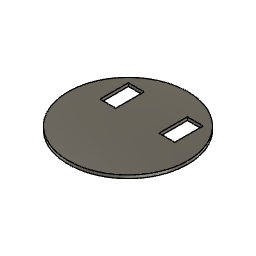
Robot assemblée v14 (Autodesk Fusion 360 archive; units mm, degrees)
design "Support robot"
Autodesk Fusion 360 part; units mm, degrees
sketch "Esquisse1" plane through (0, 0, 0) normal (0, 0, 1) x (1, 0, 0)
  circle A0 centre (0, 0) radius 95
  dimension "d1" = 190
  constraint coincident A0.centre origin
  measures "d1" diameter of A0
extrude "Extrusion1" add sketch "Esquisse1" along normal blind 5
sketch "Esquisse2" plane through (0, 0, 5) normal (0, 0, 1) x (-1, 0, 0)
  circle A0 centre (0, 0) radius 95
  line L0 (-34.3905, -60) -> (-59.3905, -60)
  line L1 (-59.3905, -60) -> (-59.3905, -15)
  line L2 (-59.3905, -15) -> (-34.3905, -15)
  line L3 (-34.3905, -15) -> (-34.3905, -60)
  line L4 (0, 95) -> (0, -95)
  line L5 (34.3905, -15) -> (34.3905, -60)
  line L6 (59.3905, -60) -> (59.3905, -15)
  line L7 (59.3905, -15) -> (34.3905, -15)
  line L8 (34.3905, -60) -> (59.3905, -60)
  dimension "d4" = 25
  dimension "d5" = 45
  constraint horizontal L0
  constraint vertical L1
  constraint horizontal L2
  constraint vertical L3
  constraint coincident A0 L4.start
  constraint coincident A0 L4.end
  constraint vertical L4
  constraint symmetric L0.start L4 L5.end
  constraint symmetric L0.end L4 L6.start
  constraint symmetric L1.end L4 L6.end
  constraint symmetric L2.end L4 L5.start
  measures "d4" distance of L0.start L0.end
  measures "d5" distance of L0.start L2.end
extrude "Extrusion2" cut sketch "Esquisse2" against normal blind 10 contours L0 L1 L2 L3 | L5 L6 L7 L8

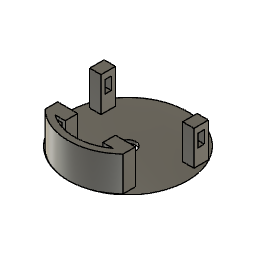
design "Socle dessus"
Autodesk Fusion 360 part; units mm, degrees
sketch "Esquisse1" plane through (0, 0, 0) normal (0, 0, 1) x (1, 0, 0)
  circle A0 centre (0, 0) radius 95
  circle A1 centre (0, 0) radius 12.5
  dimension "d1" = 190
  dimension "d2" = 25
  constraint coincident A0.centre A1.centre
  measures "d1" diameter of A0
  measures "d2" diameter of A1
extrude "Extrusion1" add sketch "Esquisse1" along normal blind 5
sketch "Esquisse2" plane through (0, 0, 5) normal (0, 0, 1) x (-1, 0, 0)
  circle A0 centre (0, 0) radius 12.5
  circle A1 centre (0, 0) radius 95
  line L0 (30, 50) -> (30, 70)
  line L1 (-65, -45) -> (-83, -45)
  line L2 (30, 70) -> (62, 70)
  line L3 (-30, 70) -> (-62, 70)
  line L4 (0, -1.75) -> (0, -22.5)
  line L5 (-65, -22) -> (-65, -45)
  arc A2 (62, 70) -> (-62, 70) centre (0, 5.62) ccw
  circle A3 centre (0, 0) radius 17.5
  arc A4 (46, 70) -> (-46, 70) centre (0, 6.9667) ccw
  line L6 (65, -22) -> (65, -45)
  line L7 (65, -45) -> (83, -45)
  line L8 (1.75, 0) -> (22.5, 0)
  line L9 (-30, 50) -> (-30, 70)
  line L10 (-62, 70) -> (-62, 50)
  line L11 (-83, -22) -> (-65, -22)
  line L12 (62, 70) -> (62, 50)
  circle A5 centre (0, 0) radius 95
  line L13 (-83, -45) -> (-83, -22)
  line L14 (83, -45) -> (83, -22)
  line L15 (62, 50) -> (30, 50)
  line L16 (-62, 50) -> (-30, 50)
  line L17 (83, -22) -> (65, -22)
  dimension "d125" = 65
  dimension "d126" = 22
  dimension "d127" = 23
  dimension "d128" = 18
  dimension "d129" = 20
  dimension "d130" = 32
  dimension "d131" = 50
  dimension "d132" = 30
  constraint horizontal L11
  constraint vertical L5
  constraint horizontal L1
  constraint vertical L13
  constraint symmetric L11.start L14.end L4
  constraint symmetric L6.start L5.start L4
  constraint symmetric L6.end L1.start L4
  constraint symmetric L1.end L7.end L4
  constraint horizontal L16
  constraint vertical L9
  constraint horizontal L3
  constraint vertical L10
  constraint symmetric L10.end L12.end L4
  constraint symmetric L9.start L0.start L4
  constraint symmetric L3.start L0.end L4
  constraint symmetric L2.end L3.end L4
  constraint tangent A2 A5
  constraint midpoint A4.start L2
  constraint midpoint A4.end L3
  measures "d125" distance of L4 L5
  measures "d126" distance of L8 L11
  measures "d127" distance of L1 L11
  measures "d128" distance of L5 L13
  measures "d129" distance of L3 L16
  measures "d130" distance of L9 L10
  measures "d131" distance of L8 L16
  measures "d132" distance of L4 L9
extrude "Extrusion2" add sketch "Esquisse2" along normal blind 55 contours L2 L3 A2 A4 | L0 L2 L12 L15 | L3 L9 L10 L16 | L1 L5 L11 L13 | L6 L7 L14 L17
fillet "Congé1" radius 95 1 edges at (-88.5711, -34.3535, 0)
sketch "Esquisse3" plane through (83, 0, 0) normal (1, 0, 0) x (0, 1, 0)
  line L0 (22, 5) -> (45, 5)
  line L1 (45, 5) -> (45, 60)
  line L2 (45, 60) -> (22, 60)
  line L3 (22, 60) -> (22, 5)
  line L4 (28.5, 50) -> (38.5, 50)
  line L5 (38.5, 50) -> (38.5, 30)
  line L6 (38.5, 30) -> (28.5, 30)
  line L7 (28.5, 30) -> (28.5, 50)
  dimension "d17" = 10
  dimension "d18" = 6.5
  dimension "d19" = 20
  constraint horizontal L4
  constraint vertical L5
  constraint horizontal L6
  constraint vertical L7
  measures "d17" distance of L5 L7
  measures "d18" distance of L3 L7
  measures "d19" distance of L4 L6
extrude "Extrusion3" cut sketch "Esquisse3" against normal blind 30 contours L4 L5 L6 L7
sketch "Esquisse4" plane through (-65, 0, 0) normal (1, 0, 0) x (0, 1, 0)
  line L0 (22, 5) -> (45, 5)
  line L1 (45, 5) -> (45, 60)
  line L2 (45, 60) -> (22, 60)
  line L3 (22, 60) -> (22, 5)
  line L4 (28.5, 50) -> (38.5, 50)
  line L5 (38.5, 50) -> (38.5, 30)
  line L6 (38.5, 30) -> (28.5, 30)
  line L7 (28.5, 30) -> (28.5, 50)
  dimension "d22" = 10
  dimension "d23" = 6.5
  dimension "d24" = 20
  dimension "d25" = 10
  constraint horizontal L4
  constraint vertical L5
  constraint horizontal L6
  constraint vertical L7
  measures "d22" distance of L5 L7
  measures "d23" distance of L3 L7
  measures "d24" distance of L4 L6
  measures "d25" distance of L2 L4
extrude "Extrusion4" cut sketch "Esquisse4" against normal blind 40 contours L4 L5 L6 L7
sketch "Esquisse5" plane through (0, -50, 0) normal (0, 1, 0) x (-1, 0, 0)
  line L0 (-62, 5) -> (-30, 5)
  line L1 (-30, 5) -> (-30, 60)
  line L2 (-30, 60) -> (-62, 60)
  line L3 (-62, 60) -> (-62, 5)
  line L4 (-50, 55) -> (-35, 55)
  line L5 (-35, 55) -> (-35, 35)
  line L6 (-35, 35) -> (-50, 35)
  line L7 (-50, 35) -> (-50, 55)
  arc A0 through (46, 60, -20) (0, 60, -35) (-46, 60, -20)
  line L8 (35, 55) -> (50, 55)
  line L9 (50, 55) -> (50, 35)
  line L10 (50, 35) -> (35, 35)
  line L11 (35, 35) -> (35, 55)
  line L12 (30, 5) -> (30, 60)
  line L13 (30, 60) -> (62, 60)
  point P0 (-30, 5)
  point P1 (30, 5)
  dimension "d29" = 5
  dimension "d30" = 15
  dimension "d31" = 20
  dimension "d32" = 5
  dimension "d33" = 15
  dimension "d34" = 5
  dimension "d35" = 20
  dimension "d37" = 5
  constraint horizontal L4
  constraint vertical L5
  constraint horizontal L6
  constraint vertical L7
  constraint horizontal L8
  constraint vertical L9
  constraint horizontal L10
  constraint vertical L11
  measures "d29" distance of L2 L4
  measures "d30" distance of L5.end L6.end
  measures "d31" distance of L4.start L6.end
  measures "d32" distance of L1 L5
  measures "d33" distance of L8.start L8.end
  measures "d34" distance of L11 L12
  measures "d35" distance of L8.end L9.end
  measures "d37" distance of L8 L13
extrude "Extrusion5" cut sketch "Esquisse5" against normal blind 20 contours L4 L5 L6 L7 | L8 L9 L10 L11

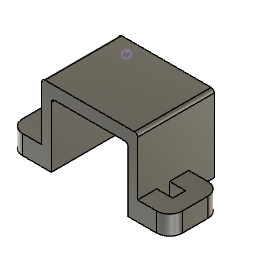
design "Support_Moteur"
Autodesk Fusion 360 part; units mm, degrees
sketch "Esquisse1" plane through (0, 0, 0) normal (0, 0, 1) x (1, 0, 0)
  line L0 (0, 0) -> (1.5, 0)
  line L1 (1.5, 0) -> (1.5, 1.2)
  line L2 (1.5, 1.2) -> (0, 1.2)
  line L3 (0, 1.2) -> (0, 0)
  dimension "d1" = 1.5
  dimension "d2" = 1.2
  constraint horizontal L0
  constraint vertical L1
  constraint horizontal L2
  constraint vertical L3
  constraint coincident L0.start L3.end
  measures "d1" distance of L0.start L0.end
  measures "d2" distance of L0.start L2.end
extrude "Extrusion1" add sketch "Esquisse1" along normal blind 1.2
sketch "Esquisse2" plane through (0, 0, 0) normal (0, 0, -1) x (1, 0, 0)
  line L0 (0, 0) -> (0, -1.2)
  line L1 (0, -1.2) -> (1.5, -1.2)
  line L2 (1.5, -1.2) -> (1.5, 0)
  line L3 (1.5, 0) -> (0, 0)
  line L4 (1.35, 0) -> (0.15, 0)
  line L5 (0.15, 0) -> (0.15, -1.2)
  line L6 (0.15, -1.2) -> (1.35, -1.2)
  line L7 (1.35, -1.2) -> (1.35, 0)
  line L8 (0.75, -1.2) -> (0.75, 0)
  dimension "d5" = 1.2
  dimension "d7" = 0.6
  constraint horizontal L4
  constraint vertical L5
  constraint horizontal L6
  constraint vertical L7
  constraint coincident L3 L4.start
  constraint midpoint L1 L8.start
  constraint midpoint L3 L8.end
  measures "d5" distance of L4.start L4.end
  measures "d7" distance of L7 L8
extrude "Extrusion2" cut sketch "Esquisse2" against normal blind 1 contours L1 L3 L4 L5 L6 L8 | L1 L3 L4 L6 L7 L8
sketch "Esquisse3" plane through (1.5, 0, 0) normal (1, 0, 0) x (0, 1, 0)
  line L0 (0, 0) -> (1.2, 0)
  line L1 (1.2, 0) -> (1.2, 1.2)
  line L2 (1.2, 1.2) -> (0, 1.2)
  line L3 (0, 1.2) -> (0, 0)
  line L4 (0, 0) -> (0.8, 0)
  line L5 (0.8, 0) -> (0.8, 0.3)
  line L6 (0.8, 0.3) -> (0, 0.3)
  line L7 (0, 0.3) -> (0, 0)
  dimension "d10" = 0.8
  dimension "d11" = 0.3
  constraint horizontal L4
  constraint vertical L5
  constraint horizontal L6
  constraint vertical L7
  constraint coincident L0.start L3.end
  measures "d10" distance of L0.start L4.end
  measures "d11" distance of L4 L6
extrude "Extrusion3" add sketch "Esquisse3" along normal blind 0.5 contours L0 L3 L4 L5 L6 L7
sketch "Esquisse4" plane through (0, 0, 0.3) normal (0, 0, 1) x (-1, 0, 0)
  line L0 (-1.5, -0.8) -> (-1.5, 0)
  line L1 (-1.5, 0) -> (-2, 0)
  line L2 (-2, 0) -> (-2, -0.8)
  line L3 (-2, -0.8) -> (-1.5, -0.8)
  line L4 (-1.5, -0.5) -> (-1.75, -0.5)
  line L5 (-1.75, -0.5) -> (-1.75, -0.3)
  line L6 (-1.75, -0.3) -> (-1.5, -0.3)
  line L7 (-1.5, -0.3) -> (-1.5, -0.5)
  line L8 (-1.5, -0.4) -> (-2, -0.4)
  dimension "d14" = 0.4
  dimension "d15" = 0.1
  dimension "d16" = 0.2
  dimension "d27" = 0.25
  constraint horizontal L4
  constraint vertical L5
  constraint horizontal L6
  constraint vertical L7
  constraint coincident L0 L4.start
  constraint coincident L0 L8.start
  constraint coincident L2 L8.end
  constraint perpendicular L2 L8
  measures "d14" distance of L3 L8
  measures "d15" distance of L6 L8
  measures "d16" distance of L4 L6
  measures "d27" distance of L5.end L6.end
extrude "Extrusion4" cut sketch "Esquisse4" against normal blind 0.5 contours L0 L4 L5 L7 L8 | L0 L5 L6 L7 L8
sketch "Esquisse5" plane through (0, 0, 0.3) normal (0, 0, 1) x (-1, 0, 0)
  line L0 (-1.75, -0.3) -> (-1.5, -0.3)
  line L1 (-1.5, -0.3) -> (-1.5, 0)
  line L2 (-1.5, 0) -> (-2, 0)
  line L3 (-2, 0) -> (-2, -0.8)
  line L4 (-2, -0.8) -> (-1.5, -0.8)
  line L5 (-1.5, -0.8) -> (-1.5, -0.5)
  line L6 (-1.5, -0.5) -> (-1.75, -0.5)
  line L7 (-1.75, -0.5) -> (-1.75, -0.3)
sketch "Esquisse6" plane through (0, 0, 0) normal (-1, 0, 0) x (0, -1, 0)
  line L0 (-1.2, 0) -> (0, 0)
  line L1 (0, 0) -> (0, 1.2)
  line L2 (0, 1.2) -> (-1.2, 1.2)
  line L3 (-1.2, 1.2) -> (-1.2, 0)
  line L4 (0, 0) -> (-0.8, 0)
  line L5 (-0.8, 0) -> (-0.8, 0.3)
  line L6 (-0.8, 0.3) -> (0, 0.3)
  line L7 (0, 0.3) -> (0, 0)
  dimension "d19" = 0.8
  dimension "d20" = 0.3
  constraint horizontal L4
  constraint vertical L5
  constraint horizontal L6
  constraint vertical L7
  constraint coincident L0.end L1.start
  measures "d19" distance of L0.end L4.end
  measures "d20" distance of L0.end L6.end
extrude "Extrusion5" add sketch "Esquisse6" along normal blind 0.5 contours L0 L1 L4 L5 L6 L7
sketch "Esquisse7" plane through (0, 0, 0.3) normal (0, 0, 1) x (-1, 0, 0)
  line L0 (0, 0) -> (0, -0.8)
  line L1 (0, -0.8) -> (0.5, -0.8)
  line L2 (0.5, -0.8) -> (0.5, 0)
  line L3 (0.5, 0) -> (0, 0)
  line L4 (0, -0.4) -> (0.5, -0.4)
  line L5 (0, -0.3) -> (0.25, -0.3)
  line L6 (0.25, -0.3) -> (0.25, -0.5)
  line L7 (0.25, -0.5) -> (0, -0.5)
  line L8 (0, -0.5) -> (0, -0.3)
  dimension "d23" = 0.25
  dimension "d24" = 0.2
  constraint midpoint L0 L4.start
  constraint midpoint L2 L4.end
  constraint horizontal L5
  constraint vertical L6
  constraint horizontal L7
  constraint vertical L8
  constraint coincident L0 L5.start
  measures "d23" distance of L5.start L5.end
  measures "d24" distance of L5.start L7.end
extrude "Extrusion6" cut sketch "Esquisse7" against normal blind 0.6 contours L0 L4 L5 L6 L8 | L0 L4 L6 L7 L8
fillet "Congé1" radius 0.2 4 edges at (2, 0, 0.15) (2, 0.8, 0.15) (-0.5, 0, 0.15) (-0.5, 0.8, 0.15)
fillet "Congé2" radius 0.05 2 edges at (1.5, 0.6, 1.2) (0, 0.6, 1.2)
fillet "Congé3" radius 0.05 2 edges at (1.35, 0.6, 1) (0.15, 0.6, 1)
scale "Echelle1" factor 10 about (0.05, 1.2, 1.2) bodies 1

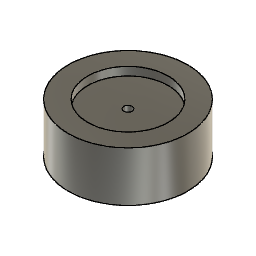
design "Roue"
Autodesk Fusion 360 part; units mm, degrees
sketch "Esquisse1" plane through (0, 0, 0) normal (0, 0, 1) x (1, 0, 0)
  circle A0 centre (0, 0) radius 2.15
  dimension "d1" = 4.3
  constraint coincident A0.centre origin
  measures "d1" diameter of A0
extrude "Extrusion1" add sketch "Esquisse1" along normal blind 1.8
sketch "Esquisse2" plane through (0, 0, 1.8) normal (0, 0, 1) x (-1, 0, 0)
  circle A0 centre (0, 0) radius 2.15
  circle A1 centre (0, 0) radius 1.45
  dimension "d4" = 2.9
  constraint concentric A0 A1
  measures "d4" diameter of A1
extrude "Extrusion2" cut sketch "Esquisse2" against normal blind 0.3 contours A1
sketch "Esquisse3" plane through (0, 0, 0) normal (0, 0, -1) x (1, 0, 0)
  circle A0 centre (0, 0) radius 2.15
  circle A1 centre (0, 0) radius 1.1
  dimension "d7" = 2.2
  constraint concentric A0 A1
  measures "d7" diameter of A1
extrude "Extrusion3" cut sketch "Esquisse3" against normal blind 0.5 contours A1
sketch "Esquisse4" plane through (0, 0, 1.5) normal (0, 0, 1) x (-1, 0, 0)
  circle A0 centre (0, 0) radius 1.45
  circle A1 centre (0, 0) radius 0.15
  dimension "d10" = 0.3
  constraint concentric A0 A1
  measures "d10" diameter of A1
extrude "Extrusion4" cut sketch "Esquisse4" against normal blind 3.8 contours A1
scale "Echelle1" factor 10 about (1.45, 0, 1.8) bodies 1

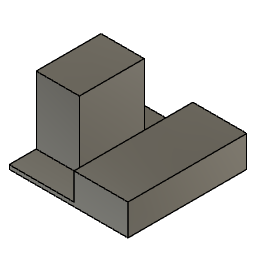
design "MotorDriver"
Autodesk Fusion 360 part; units mm, degrees
sketch "Esquisse1" plane through (0, 0, 0) normal (0, 0, 1) x (1, 0, 0)
  line L0 (0, 0) -> (4.4, 0)
  line L1 (4.4, 0) -> (4.4, 4.4)
  line L2 (4.4, 4.4) -> (0, 4.4)
  line L3 (0, 4.4) -> (0, 0)
  dimension "d1" = 4.4
  dimension "d2" = 4.4
  constraint horizontal L0
  constraint vertical L1
  constraint horizontal L2
  constraint vertical L3
  constraint coincident L0.start L3.end
  measures "d1" distance of L0.start L0.end
  measures "d2" distance of L0.start L2.end
extrude "Extrusion1" add sketch "Esquisse1" along normal blind 0.15
sketch "Esquisse2" plane through (0, 0, 0.15) normal (0, 0, 1) x (-1, 0, 0)
  line L0 (0, -4.4) -> (0, 0)
  line L1 (0, 0) -> (-4.4, 0)
  line L2 (-4.4, 0) -> (-4.4, -4.4)
  line L3 (-4.4, -4.4) -> (0, -4.4)
  line L4 (-4.4, 0) -> (-2.4, 0)
  line L5 (-2.4, 0) -> (-2.4, -4.4)
  line L6 (-2.4, -4.4) -> (-4.4, -4.4)
  line L7 (-4.4, -4.4) -> (-4.4, 0)
  dimension "d5" = 2
  constraint horizontal L4
  constraint vertical L5
  constraint horizontal L6
  constraint vertical L7
  constraint coincident L3 L5.end
  constraint coincident L1.end L2.start
  measures "d5" distance of L1.end L4.end
extrude "Extrusion2" add sketch "Esquisse2" along normal blind 1 contours L1 L2 L3 L4 L5 L6 L7
sketch "Esquisse3" plane through (0, 0, 0.15) normal (0, 0, 1) x (-1, 0, 0)
  line L0 (-2.4, 0) -> (-2.4, -4.4)
  line L1 (-2.4, -4.4) -> (0, -4.4)
  line L2 (0, -4.4) -> (0, 0)
  line L3 (0, 0) -> (-2.4, 0)
  line L4 (0, -3.4) -> (-1.6, -3.4)
  line L5 (-1.6, -3.4) -> (-1.6, -1)
  line L6 (-1.6, -1) -> (0, -1)
  line L7 (0, -1) -> (0, -3.4)
  dimension "d8" = 1.6
  dimension "d9" = 2.4
  dimension "d11" = 1
  constraint horizontal L4
  constraint vertical L5
  constraint horizontal L6
  constraint vertical L7
  constraint coincident L2 L4.start
  measures "d8" distance of L4.start L4.end
  measures "d9" distance of L4.start L6.end
  measures "d11" distance of L3 L6
extrude "Extrusion3" add sketch "Esquisse3" along normal blind 2.5 contours L2 L4 L5 L6 L7
scale "Echelle1" factor 10 about (0, 3.4, 2.65) bodies 1

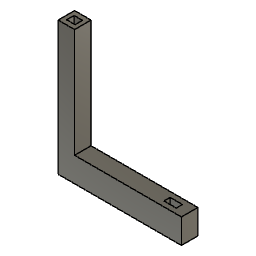
design "Bras moteur boule"
Autodesk Fusion 360 part; units mm, degrees
sketch "Esquisse1" plane through (0, 0, 0) normal (0, 0, 1) x (1, 0, 0)
  line L0 (0, 0) -> (8, 0)
  line L1 (8, 0) -> (8, 8)
  line L2 (8, 8) -> (0, 8)
  line L3 (0, 8) -> (0, 0)
  dimension "d1" = 8
  dimension "d2" = 8
  constraint horizontal L0
  constraint vertical L1
  constraint horizontal L2
  constraint vertical L3
  constraint coincident L0.start L3.end
  measures "d1" distance of L1.end L2.end
  measures "d2" distance of L0.start L2.end
extrude "Extrusion1" add sketch "Esquisse1" along normal blind 65
sketch "Esquisse8" plane through (0, 0, 65) normal (0, 0, 1) x (-1, 0, 0)
  line L0 (0, -8) -> (0, 0)
  line L1 (0, 0) -> (-8, 0)
  line L2 (-8, 0) -> (-8, -8)
  line L3 (-8, -8) -> (0, -8)
  line L4 (0, -4) -> (-8, -4)
  line L5 (-1.95, -4) -> (-6.05, -4)
  line L6 (-6.05, -4) -> (-6.05, -5.8)
  line L7 (-6.05, -5.8) -> (-1.95, -5.8)
  line L8 (-1.95, -5.8) -> (-1.95, -4)
  line L9 (-4, -8) -> (-4, 0)
  line L10 (-1.95, -2.2) -> (-1.95, -4)
  line L11 (-6.05, -2.2) -> (-1.95, -2.2)
  line L12 (-6.05, -4) -> (-6.05, -2.2)
  dimension "d41" = 4.1
  dimension "d42" = 2.05
  dimension "d43" = 1.8
  constraint midpoint L0 L4.start
  constraint midpoint L2 L4.end
  constraint horizontal L5
  constraint vertical L6
  constraint horizontal L7
  constraint vertical L8
  constraint coincident L4 L5.start
  constraint midpoint L3 L9.start
  constraint midpoint L1 L9.end
  constraint symmetric L8.end L5 L10.end
  constraint symmetric L6.start L5 L12.start
  constraint symmetric L6.end L5 L11.start
  constraint symmetric L7.end L5 L10.start
  measures "d41" distance of L6 L8
  measures "d42" distance of L8 L9
  measures "d43" distance of L5.start L7.end
extrude "Extrusion8" cut sketch "Esquisse8" against normal blind 6 contours L4 L5 L7 L8 L9 | L4 L5 L9 L10 L11 | L4 L5 L6 L7 L9 | L4 L5 L9 L11 L12
sketch "Esquisse9" plane through (8, 0, 0) normal (1, 0, 0) x (0, 1, 0)
  line L0 (0, 0) -> (8, 0)
  line L1 (8, 0) -> (8, 65)
  line L2 (8, 65) -> (0, 65)
  line L3 (0, 65) -> (0, 0)
  line L4 (0, 0) -> (8, 0)
  line L5 (8, 0) -> (8, 12)
  line L6 (8, 12) -> (0, 12)
  line L7 (0, 12) -> (0, 0)
  dimension "d46" = 12
  constraint horizontal L4
  constraint vertical L5
  constraint horizontal L6
  constraint vertical L7
  constraint coincident L1 L5.end
  constraint coincident L0.start L3.end
  measures "d46" distance of L4 L6
extrude "Extrusion9" add sketch "Esquisse9" along normal blind 52 contours L0 L1 L3 L4 L5 L6 L7
sketch "Esquisse10" plane through (0, 0, 12) normal (0, 0, 1) x (-1, 0, 0)
  line L0 (-8, -8) -> (-8, 0)
  line L1 (-8, 0) -> (-60, 0)
  line L2 (-60, 0) -> (-60, -8)
  line L3 (-60, -8) -> (-8, -8)
  line L4 (-55, -5.5) -> (-49, -5.5)
  line L5 (-49, -5.5) -> (-49, -2.5)
  line L6 (-49, -2.5) -> (-55, -2.5)
  line L7 (-55, -2.5) -> (-55, -5.5)
  dimension "d49" = 2.5
  dimension "d50" = 2.5
  dimension "d51" = 5
  dimension "d52" = 6
  constraint horizontal L4
  constraint vertical L5
  constraint horizontal L6
  constraint vertical L7
  measures "d49" distance of L3 L4
  measures "d50" distance of L1 L6
  measures "d51" distance of L2 L7
  measures "d52" distance of L5 L7
extrude "Extrusion10" cut sketch "Esquisse10" against normal blind 23 contours L4 L5 L6 L7

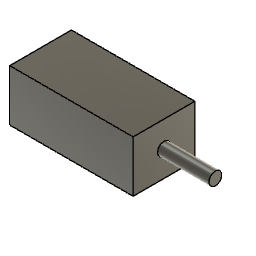
design "Moteur"
Autodesk Fusion 360 part; units mm, degrees
sketch "Esquisse1" plane through (0, 0, 0) normal (0, 0, 1) x (1, 0, 0)
  line L0 (0, 0) -> (2.4, 0)
  line L1 (2.4, 0) -> (2.4, 1.2)
  line L2 (2.4, 1.2) -> (0, 1.2)
  line L3 (0, 1.2) -> (0, 0)
  dimension "d1" = 2.4
  dimension "d2" = 1.2
  constraint horizontal L0
  constraint vertical L1
  constraint horizontal L2
  constraint vertical L3
  constraint coincident L0.start L3.end
  measures "d1" distance of L0.start L0.end
  measures "d2" distance of L0.end L2
extrude "Extrusion1" add sketch "Esquisse1" along normal blind 1
sketch "Esquisse2" plane through (2.4, 0, 0) normal (1, 0, 0) x (0, 1, 0)
  line L0 (0, 0) -> (1.2, 0)
  line L1 (1.2, 0) -> (1.2, 1)
  line L2 (1.2, 1) -> (0, 1)
  line L3 (0, 1) -> (0, 0)
  circle A0 centre (0.6, 0.5) radius 0.125
  dimension "d5" = 0.25
  measures "d5" diameter of A0
extrude "Extrusion2" add sketch "Esquisse2" along normal blind 1 contours A0
scale "Echelle1" factor 10 about (0, 1.2, 1) bodies 1

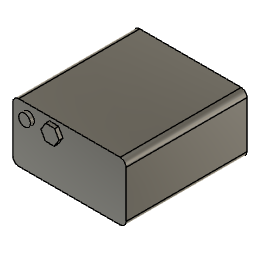
design "Bloc pile 12V"
Autodesk Fusion 360 part; units mm, degrees
sketch "Esquisse1" plane through (0, 0, 0) normal (0, 0, 1) x (1, 0, 0)
  line L0 (0, 0) -> (58, 0)
  line L1 (58, 0) -> (58, 62)
  line L2 (58, 62) -> (0, 62)
  line L3 (0, 62) -> (0, 0)
  dimension "d1" = 58
  dimension "d2" = 62
  constraint horizontal L0
  constraint vertical L1
  constraint horizontal L2
  constraint vertical L3
  constraint coincident L0.start L3.end
  measures "d1" distance of L0.start L0.end
  measures "d2" distance of L0.start L2.end
extrude "Extrusion1" add sketch "Esquisse1" along normal blind 30
fillet "Congé1" radius 3 4 edges at (58, 31, 30) (58, 31, 0) (0, 31, 30) (0, 31, 0)
sketch "Esquisse2" plane through (0, 0, 0) normal (0, -1, 0) x (1, 0, 0)
  arc A0 (0, 3) -> (3, 0) centre (3, 3) ccw
  line L0 (3, 0) -> (55, 0)
  arc A1 (55, 0) -> (58, 3) centre (55, 3) ccw
  line L1 (58, 3) -> (58, 27)
  arc A2 (58, 27) -> (55, 30) centre (55, 27) ccw
  line L2 (55, 30) -> (3, 30)
  arc A3 (3, 30) -> (0, 27) centre (3, 27) ccw
  line L3 (0, 27) -> (0, 3)
  circle A4 centre (8, 24) radius 3
  dimension "d7" = 6
  dimension "d8" = 6
  dimension "d9" = 8
  measures "d7" diameter of A4
  measures "d8" distance of L2 A4.centre
  measures "d9" distance of L3 A4.centre
sketch "Esquisse3" plane through (0, 0, 0) normal (0, -1, 0) x (1, 0, 0)
  line L0 (18.832, 28.0784) -> (16.384, 24.1616)
  line L1 (16.384, 24.1616) -> (18.552, 20.0833)
  line L2 (18.552, 20.0833) -> (23.168, 19.9216)
  line L3 (23.168, 19.9216) -> (25.616, 23.8384)
  line L4 (25.616, 23.8384) -> (23.448, 27.9167)
  line L5 (23.448, 27.9167) -> (18.832, 28.0784)
  line L6 (55, 30) -> (3, 30)
  line L7 (0, 27) -> (0, 3)
  point P0 (21, 24)
  dimension "d10" = 8
  dimension "d11" = 6
  dimension "d12" = 21
  measures "d10" distance of L2 L5
  measures "d11" distance of P0 L6
  measures "d12" distance of P0 L7
extrude "Extrusion2" add sketch "Esquisse2" sketch "Esquisse3" along normal blind 2 contours A4 of sketch 2

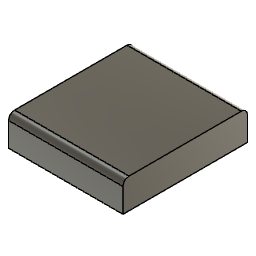
design "Bloc Pile 6v"
Autodesk Fusion 360 part; units mm, degrees
sketch "Esquisse1" plane through (0, 0, 0) normal (0, 0, 1) x (1, 0, 0)
  line L0 (0, 0) -> (57, 0)
  line L1 (57, 0) -> (57, 62)
  line L2 (57, 62) -> (0, 62)
  line L3 (0, 62) -> (0, 0)
  dimension "d1" = 57
  dimension "d2" = 62
  constraint horizontal L0
  constraint vertical L1
  constraint horizontal L2
  constraint vertical L3
  constraint coincident L0.start L3.end
  measures "d1" distance of L0.start L0.end
  measures "d2" distance of L0.start L2.end
extrude "Extrusion1" add sketch "Esquisse1" along normal blind 15
fillet "Congé1" radius 3 2 edges at (28.5, 62, 15) (28.5, 0, 15)

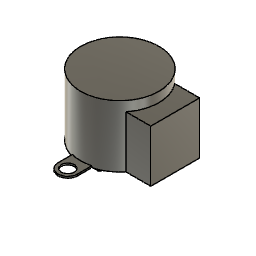
design "Moteur_Boule"
Autodesk Fusion 360 part; units mm, degrees
sketch "Esquisse1" plane through (0, 0, 0) normal (0, 0, 1) x (1, 0, 0)
  circle A0 centre (0, 0) radius 12
  line L0 (9, 0) -> (17, 0)
  line L1 (17, -7.5) -> (9, -7.5)
  line L2 (9, -7.5) -> (9, 7.5)
  line L3 (9, 7.5) -> (17, 7.5)
  line L4 (17, 7.5) -> (17, -7.5)
  dimension "d1" = 24
  dimension "d3" = 8
  dimension "d4" = 17
  dimension "d5" = 15
  dimension "d8" = 7.5
  dimension "d9" = 8
  constraint coincident A0.centre origin
  constraint horizontal L0
  constraint horizontal L1
  constraint vertical L2
  constraint horizontal L3
  constraint vertical L4
  constraint collinear A0.centre L0.start L0.end
  constraint collinear L0.end L1.start L3.end
  measures "d1" diameter of A0
  measures "d3" distance of L0.start L0.end
  measures "d4" distance of A0.centre L0.end
  measures "d5" distance of L1 L3
  measures "d8" distance of L0 L1
  measures "d9" distance of L2.end L3.end
extrude "Extrusion1" add sketch "Esquisse1" along normal blind 16
sketch "Esquisse2" plane through (0, 0, 16) normal (0, 0, 1) x (-1, 0, 0)
  arc A0 (-9.3675, -7.5) -> (-9.3675, 7.5) centre (0, 0) ccw
  line L0 (-9.3675, 7.5) -> (-17, 7.5)
  line L1 (-17, 7.5) -> (-17, -7.5)
  line L2 (-17, -7.5) -> (-9.3675, -7.5)
  circle A1 centre (0, 0) radius 12
  constraint concentric A0 A1
extrude "Extrusion2" add sketch "Esquisse2" along normal blind 3 contours A0 A1
sketch "Esquisse5" plane through (0, 0, 0) normal (0, 0, -1) x (1, 0, 0)
  arc A0 (9.3675, 7.5) -> (9.3675, -7.5) centre (0, 0) ccw
  line L0 (9.3675, -7.5) -> (17, -7.5)
  line L1 (17, -7.5) -> (17, 7.5)
  line L2 (17, 7.5) -> (9.3675, 7.5)
  circle A1 centre (0, 16) radius 2
  line L3 (0, 0) -> (12, 0)
  circle A2 centre (0, 0) radius 12
  line L4 (3, 16) -> (3, 11.619)
  line L5 (0, 0) -> (0, 19)
  arc A3 (-3, -16) -> (0, -19) centre (0, -16) ccw
  line L6 (3, -16) -> (3, -11.619)
  circle A4 centre (0, -16) radius 2
  line L7 (-3, 16) -> (-3, 11.619)
  arc A5 (0, -19) -> (3, -16) centre (0, -16) ccw
  arc A6 (0, 19) -> (-3, 16) centre (0, 16) ccw
  line L8 (-3, 16) -> (3, 16)
  arc A7 (3, 16) -> (0, 19) centre (0, 16) ccw
  line L9 (-3, -16) -> (-3, -11.619)
  point P0 (0, 12)
  dimension "d27" = 19
  dimension "d28" = 4
  dimension "d29" = 24
  dimension "d30" = 3
  constraint coincident A0.centre L3.start
  constraint vertical L5
  constraint coincident A1.centre L5
  constraint coincident P0 L5
  constraint perpendicular L3 L5
  constraint coincident A1.centre A6.centre
  constraint perpendicular L5 L8
  constraint coincident L4.end A2
  constraint tangent L4 A7
  constraint coincident L7.end A2
  constraint tangent L7 A6
  constraint perpendicular L7 L8
  constraint symmetric A3.end L5.end L3
  constraint symmetric A1 L3 A4
  constraint symmetric L6.start L4.start L3
  constraint symmetric L3 A5 A7
  constraint symmetric A3.start L7.start L3
  constraint symmetric L3 A3 A6
  constraint symmetric L4.end L6.end L3
  constraint symmetric L7.end L9.end L3
  measures "d27" distance of A0.centre L5.end
  measures "d28" diameter of A1
  measures "d29" diameter of A2
  measures "d30" distance of L8 A7
extrude "Extrusion4" add sketch "Esquisse5" against normal blind 0.5 contours A0 A1 A2 L4 L5 L8 | A0 A1 A2 L5 L7 L8 | A1 L5 L8 A7 | A1 L5 A6 L8 | A0 A2 A3 L6 A5 L9
sketch "Esquisse6" plane through (0, 0, 0) normal (0, 0, -1) x (1, 0, 0)
  circle A0 centre (0, -16) radius 2
  circle A1 centre (0, 16) radius 2
  arc A2 (3, -11.619) -> (9.3675, -7.5) centre (0, 0) ccw
  line L0 (9.3675, -7.5) -> (17, -7.5)
  line L1 (17, -7.5) -> (17, 7.5)
  line L2 (17, 7.5) -> (9.3675, 7.5)
  arc A3 (9.3675, 7.5) -> (3, 11.619) centre (0, 0) ccw
  line L3 (3, 11.619) -> (3, 16)
  arc A4 (3, 16) -> (-3, 16) centre (0, 16) ccw
  line L4 (-3, 16) -> (-3, 11.619)
  arc A5 (-3, 11.619) -> (-3, -11.619) centre (0, 0) ccw
  line L5 (-3, -11.619) -> (-3, -16)
  arc A6 (-3, -16) -> (3, -16) centre (0, -16) ccw
  line L6 (3, -16) -> (3, -11.619)
  circle A7 centre (-7, 0) radius 4
  line L7 (-7, 0) -> (-12, 0)
  dimension "d33" = 8
  dimension "d34" = 5
  constraint coincident A7.centre L7.start
  constraint midpoint A5 L7.end
  constraint horizontal L7
  measures "d33" diameter of A7
  measures "d34" distance of A7.centre L7.end
extrude "Extrusion5" add sketch "Esquisse6" along normal blind 1 contours A7
sketch "Esquisse7" plane through (0, 0, -1) normal (0, 0, -1) x (1, 0, 0)
  circle A0 centre (-7, 0) radius 4
  circle A1 centre (-7, 0) radius 2.5
  dimension "d37" = 5
  constraint concentric A0 A1
  measures "d37" diameter of A1
extrude "Extrusion6" add sketch "Esquisse7" along normal blind 9 contours A1
sketch "Esquisse8" plane through (0, 0, -10) normal (0, 0, -1) x (1, 0, 0)
  circle A0 centre (-7, 0) radius 2.5
  line L0 (-7, 0) -> (-9.5, 0)
  line L1 (-7, 0) -> (-4.5, 0)
  line L2 (-9, 0) -> (-5, 0)
  line L3 (-5, 0) -> (-5, 1.5)
  line L4 (-5, 1.5) -> (-9, 1.5)
  line L5 (-9, 1.5) -> (-9, 0)
  line L6 (-5, -1.5) -> (-9, -1.5)
  line L7 (-9, -1.5) -> (-9, 0)
  line L8 (-5, 0) -> (-5, -1.5)
  dimension "d43" = 4
  dimension "d44" = 1.5
  dimension "d45" = 2
  constraint coincident A0.centre L0.start
  constraint coincident A0 L0.end
  constraint horizontal L0
  constraint coincident A0 L1.end
  constraint parallel L0 L1
  constraint horizontal L2
  constraint vertical L3
  constraint horizontal L4
  constraint vertical L5
  constraint coincident L0 L2.start
  constraint symmetric L5.end L2 L7.end
  constraint symmetric L3.start L2 L8.start
  constraint symmetric L3.end L2 L6.start
  constraint symmetric L4.end L2 L6.end
  measures "d43" distance of L3.end L4.end
  measures "d44" distance of L1 L4
  measures "d45" distance of A0.centre L5
extrude "Extrusion7" cut sketch "Esquisse8" against normal blind 6 contours A0 L4 | A0 L6

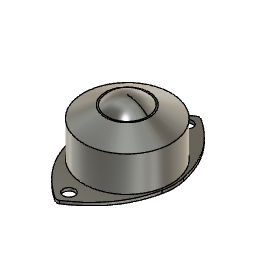
design "Roue Pivot"
Autodesk Fusion 360 part; units mm, degrees
sketch "Esquisse1" plane through (0, 0, 0) normal (0, 0, 1) x (1, 0, 0)
  circle A0 centre (0, 0) radius 16
  line L0 (0, 25) -> (0, -25)
  line L1 (0, 16) -> (0, 25)
  circle A1 centre (0, 20.5) radius 2
  spline S0 degree 5 poles (-15.998, 0.25) (-15.7389, 1.9932) (-15.1133, 5.2622) (-13.8531, 9.5141) (-11.6152, 14.0579) (-8.1767, 18.4749) (-5.0788, 21.3679) (-2.5998, 23.2801) (-0.8781, 24.445) (0, 25) knots 0 0 0 0 0 0 0.2 0.4 0.6 0.8 1 1 1 1 1 1
  line L2 (-16.6171, -3.9145) -> (-15.379, 4.4145)
  spline S1 degree 5 poles (15.998, 0.25) (15.7389, 1.9932) (15.1133, 5.2622) (13.8531, 9.5141) (11.6152, 14.0579) (8.1767, 18.4749) (5.0788, 21.3679) (2.5998, 23.2801) (0.8781, 24.445) (0, 25) knots 0 0 0 0 0 0 0.2 0.4 0.6 0.8 1 1 1 1 1 1
  line L3 (-2.0948, 23.676) -> (2.0948, 26.324)
  line L4 (16.6171, -3.9145) -> (15.379, 4.4145)
  line L5 (2.0948, 23.676) -> (-2.0948, 26.324)
  line L6 (-15.998, 0.25) -> (15.998, 0.25)
  spline S2 degree 5 poles (-15.998, 0.25) (-15.7389, -1.4932) (-15.1133, -4.7622) (-13.8531, -9.0141) (-11.6152, -13.5579) (-8.1767, -17.9749) (-5.0788, -20.8679) (-2.5998, -22.7801) (-0.8781, -23.945) (0, -24.5) knots 0 0 0 0 0 0 0.2 0.4 0.6 0.8 1 1 1 1 1 1
  line L7 (-16.6171, 4.4145) -> (-15.379, -3.9145)
  line L8 (-2.0948, -23.176) -> (2.0948, -25.824)
  spline S3 degree 5 poles (15.998, 0.25) (15.7389, -1.4932) (15.1133, -4.7622) (13.8531, -9.0141) (11.6152, -13.5579) (8.1767, -17.9749) (5.0788, -20.8679) (2.5998, -22.7801) (0.8781, -23.945) (0, -24.5) knots 0 0 0 0 0 0 0.2 0.4 0.6 0.8 1 1 1 1 1 1
  line L9 (16.6171, 4.4145) -> (15.379, -3.9145)
  line L10 (2.0948, -23.176) -> (-2.0948, -25.824)
  circle A2 centre (0, -20) radius 2
  point P0 (0, 16)
  dimension "d1" = 32
  dimension "d2" = 50
  dimension "d3" = 25
  dimension "d4" = 4
  constraint coincident A0.centre origin
  constraint vertical L0
  constraint coincident A0 P0
  constraint coincident L0 P0
  constraint midpoint L1 A1.centre
  constraint coincident A0 S0.start
  constraint midpoint S0.start L2
  constraint coincident A0 L2.end
  constraint midpoint L0.start L3
  constraint symmetric L1.end L0 S0.end
  constraint symmetric L0 P0 L1.start
  constraint symmetric L0 S0.start S1.start
  constraint symmetric L0 L2.start L4.start
  constraint symmetric L0 L2.end L4.end
  constraint symmetric L0 L3.start L5.start
  constraint symmetric L0 L3.end L5.end
  constraint symmetric L0.start L6 S2.end
  constraint symmetric A1 L6 A2
  constraint symmetric S0.start L6 S2.start
  constraint symmetric L2.start L6 L7.start
  constraint symmetric L2.end L6 L7.end
  constraint symmetric S1.start L6 S3.start
  constraint symmetric L3.start L6 L8.start
  constraint symmetric L3.end L6 L8.end
  constraint symmetric L4.start L6 L9.start
  constraint symmetric L4.end L6 L9.end
  constraint symmetric L5.start L6 L10.start
  constraint symmetric L5.end L6 L10.end
  measures "d1" diameter of A0
  measures "d2" distance of L0.start L0.end
  measures "d3" distance of A0.centre L0.start
  measures "d4" diameter of A1
extrude "Extrusion1" add sketch "Esquisse1" along normal blind 1 contours A0 L0 S1 L6 | A0 L0 L6 S3 | A0 L0 S3 A2 | A0 L0 L1 A1 S1 | A0 L0 S0 L6 | A0 L0 L6 S2 | A0 L0 S2 A2 | A0 L0 L1 A1 S0
sketch "Esquisse2" plane through (0, 0, 1) normal (0, 0, 1) x (-1, 0, 0)
  circle A0 centre (0, -20.5) radius 2
  circle A1 centre (0, 20) radius 2
  spline S0 degree 5 poles (15.998, -0.25) (15.7389, 1.4932) (15.1133, 4.7622) (13.8531, 9.0141) (11.6152, 13.5579) (8.1767, 17.9749) (5.0788, 20.8679) (2.5998, 22.7801) (0.8781, 23.945) (0, 24.5) knots 0 0 0 0 0 0 0.2 0.4 0.6 0.8 1 1 1 1 1 1
  spline S1 degree 5 poles (0, 24.5) (-0.8781, 23.945) (-2.5998, 22.7801) (-5.0788, 20.8679) (-8.1767, 17.9749) (-11.6152, 13.5579) (-13.8531, 9.0141) (-15.1133, 4.7622) (-15.7389, 1.4932) (-15.998, -0.25) knots -1 -1 -1 -1 -1 -1 -0.8 -0.6 -0.4 -0.2 0 0 0 0 0 0
  spline S2 degree 5 poles (-15.998, -0.25) (-15.7389, -1.9932) (-15.1133, -5.2622) (-13.8531, -9.5141) (-11.6152, -14.0579) (-8.1767, -18.4749) (-5.0788, -21.3679) (-2.5998, -23.2801) (-0.8781, -24.445) (0, -25) knots 0 0 0 0 0 0 0.2 0.4 0.6 0.8 1 1 1 1 1 1
  spline S3 degree 5 poles (0, -25) (0.8781, -24.445) (2.5998, -23.2801) (5.0788, -21.3679) (8.1767, -18.4749) (11.6152, -14.0579) (13.8531, -9.5141) (15.1133, -5.2622) (15.7389, -1.9932) (15.998, -0.25) knots -1 -1 -1 -1 -1 -1 -0.8 -0.6 -0.4 -0.2 0 0 0 0 0 0
  circle A2 centre (0, 0) radius 15
  dimension "d7" = 30
  constraint coincident A2.centre origin
  measures "d7" diameter of A2
extrude "Extrusion2" add sketch "Esquisse2" along normal blind 12 contours A2
fillet "Congé1" radius 1.5 2 edges at (0, -24.5, 0.5) (0, 25, 0.5)
sketch "Esquisse4" plane through (0, 0, 0) normal (0, 1, 0) x (1, 0, 0)
  line L0 (0, -13) -> (0, -17)
  line L1 (0, -17) -> (7.5, -17)
  line L2 (7.5, -17) -> (15, -13)
  line L3 (0, -13) -> (15, -13)
  dimension "d15" = 4
  dimension "d16" = 7.5
  constraint vertical L0
  constraint perpendicular L0 L1
  constraint perpendicular L0 L3
  measures "d15" distance of L0.start L0.end
  measures "d16" distance of L0.end L1.end
revolve "Révolution1" add sketch "Esquisse4" angle 360 about axis through (0, 0, 13) along (0, 0, 1)
sketch "Esquisse5" plane through (0, 0, 0) normal (0, 1, 0) x (1, 0, 0)
  line L0 (0, -17) -> (0, -20)
  spline S0 degree 5 poles (0, -20) (0.408, -20) (1.1867, -19.965) (2.2427, -19.8075) (3.4576, -19.4165) (4.7621, -18.7269) (5.7006, -18.0768) (6.3647, -17.5519) (6.791, -17.1866) (7, -17) knots 0 0 0 0 0 0 0.2 0.4 0.6 0.8 1 1 1 1 1 1
  line L1 (-1, -20) -> (1, -20)
  line L2 (0, -17) -> (7, -17)
  dimension "d18" = 20
  dimension "d19" = 7
  constraint vertical L0
  constraint midpoint L0.end L1
  constraint perpendicular L0 L2
  measures "d18" distance of origin L0.end
  measures "d19" distance of L0 S0.end
revolve "Révolution2" add sketch "Esquisse5" angle 360 about axis through (0, 0, 17) along (0, 0, 1)
fillet "Congé2" radius 16.5 2 edges at (15.998, 0.25, 0.5) (-15.998, 0.25, 0.5)

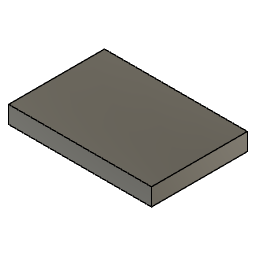
design "BreadBord Commande"
Autodesk Fusion 360 part; units mm, degrees
sketch "Esquisse1" plane through (0, 0, 0) normal (0, 0, 1) x (1, 0, 0)
  line L0 (0, 0) -> (82, 0)
  line L1 (82, 0) -> (82, 55)
  line L2 (82, 55) -> (0, 55)
  line L3 (0, 55) -> (0, 0)
  dimension "d1" = 82
  dimension "d2" = 55
  constraint horizontal L0
  constraint vertical L1
  constraint horizontal L2
  constraint vertical L3
  constraint coincident L0.start L3.end
  measures "d1" distance of L0.start L0.end
  measures "d2" distance of L0.start L2.end
extrude "Extrusion1" add sketch "Esquisse1" along normal blind 10

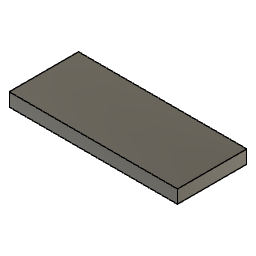
design "Raspberry Pi Pico"
Autodesk Fusion 360 part; units mm, degrees
sketch "Esquisse1" plane through (0, 0, 0) normal (0, 0, 1) x (1, 0, 0)
  line L0 (0, 0) -> (51, 0)
  line L1 (51, 0) -> (51, 21)
  line L2 (51, 21) -> (0, 21)
  line L3 (0, 21) -> (0, 0)
  dimension "d1" = 51
  dimension "d2" = 21
  constraint horizontal L0
  constraint vertical L1
  constraint horizontal L2
  constraint vertical L3
  constraint coincident L0.start L3.end
  measures "d1" distance of L0.start L0.end
  measures "d2" distance of L0.start L2.end
extrude "Extrusion1" add sketch "Esquisse1" along normal blind 4
